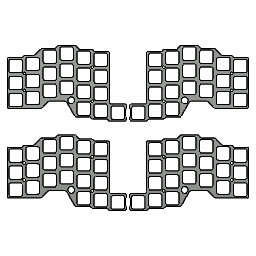
mriya-spacer-fdm-v.1.01 (Autodesk Fusion 360 design; units mm, degrees)
Autodesk Fusion 360 part; units mm, degrees
note: some values were not read from the file. Set by a fixed rule: which sketch regions a step uses.
(part 1 of 2)
sketch "mriya-spacer-fdm" plane through (0, 0, 0) normal (0, 0, 1) x (1, 0, 0)
  arc A0 (-5.2, 2.5932) -> (-4.4, 3.3932) centre (-5.2, 3.3932) ccw construction
  line L0 (-2.1, 1.9932) -> (-2.1, 37.3932) construction
  arc A1 (-3.6, 0.4932) -> (-2.1, 1.9932) centre (-3.6, 1.9932) ccw construction
  line L1 (-36.6, 37.8932) -> (-24.2, 37.8932) construction
  line L2 (-36.6, 23.8932) -> (-24.2, 23.8932) construction
  line L3 (-36.6, 18.8932) -> (-24.2, 18.8932) construction
  line L4 (-36.6, 4.8932) -> (-24.2, 4.8932) construction
  arc A2 (-67.7517, 20.7608) -> (-71.2344, 22.7932) centre (-71.2344, 18.793) ccw construction
  line L5 (-39.0716, 2.7932) -> (-24.0284, 2.7932) construction
  line L6 (-36.6, 42.8932) -> (-24.2, 42.8932) construction
  arc A3 (-56.4, 7.9932) -> (-55.6, 7.1932) centre (-55.6, 7.9932) ccw construction
  arc A4 (-36.6, 18.8932) -> (-37.4, 18.0932) centre (-36.6, 18.0932) ccw construction
  line L7 (-37.4, 18.0932) -> (-37.4, 5.6932) construction
  arc A5 (-40.4858, 3.379) -> (-39.0716, 2.7932) centre (-39.0716, 4.7932) ccw construction
  circle A6 centre (-39.9, 22.5432) radius 1.7
  arc A7 (-20.7, 39.1932) -> (-19.7, 38.1932) centre (-19.7, 39.1932) ccw construction
  line L8 (-3.6, 0.4932) -> (-20.0716, 0.4932) construction
  arc A8 (-17.6, 16.5932) -> (-18.4, 15.7932) centre (-17.6, 15.7932) ccw construction
  line L9 (-17.6, 16.5932) -> (-5.2, 16.5932) construction
  arc A9 (-18.4, 3.3932) -> (-17.6, 2.5932) centre (-17.6, 3.3932) ccw construction
  arc A10 (-2.1, 37.3932) -> (-2.9, 38.1932) centre (-2.9, 37.3932) ccw construction
  arc A11 (-4.4, 15.7932) -> (-5.2, 16.5932) centre (-5.2, 15.7932) ccw construction
  line L10 (-19.7, 38.1932) -> (-2.9, 38.1932) construction
  line L11 (-18.4, 15.7932) -> (-18.4, 3.3932) construction
  line L12 (-17.6, 2.5932) -> (-5.2, 2.5932) construction
  line L13 (-2.8, 14.0932) -> (-2.8, 5.0932)
  line L14 (-4.4, 15.7932) -> (-4.4, 3.3932) construction
  arc A12 (-24.2, 4.8932) -> (-23.4, 5.6932) centre (-24.2, 5.6932) ccw construction
  line L15 (-56.4, 39.3932) -> (-56.4, 26.9932) construction
  line L16 (-42.4, 39.3932) -> (-42.4, 26.9932) construction
  line L17 (-55.6, 40.1932) -> (-43.2, 40.1932) construction
  arc A13 (-36.6, 37.8932) -> (-37.4, 37.0932) centre (-36.6, 37.0932) ccw construction
  arc A14 (-62.2, 30.6932) -> (-61.4, 31.4932) centre (-62.2, 31.4932) ccw construction
  line L18 (-61.4, 43.8932) -> (-61.4, 31.4932) construction
  line L19 (-55.6, 26.1932) -> (-43.2, 26.1932) construction
  line L20 (-55.6, 45.1932) -> (-43.2, 45.1932) construction
  arc A15 (-43.2, 26.1932) -> (-42.4, 26.9932) centre (-43.2, 26.9932) ccw construction
  line L21 (-36.6, 56.8932) -> (-24.2, 56.8932) construction
  arc A16 (-23.4, 56.0932) -> (-24.2, 56.8932) centre (-24.2, 56.0932) ccw construction
  arc A17 (-62.2, 49.6932) -> (-61.4, 50.4932) centre (-62.2, 50.4932) ccw construction
  arc A18 (-36.6, 56.8932) -> (-37.4, 56.0932) centre (-36.6, 56.0932) ccw construction
  arc A19 (-36.6, 75.8932) -> (-37.4, 75.0932) centre (-36.6, 75.0932) ccw construction
  arc A20 (-43.2, 64.1932) -> (-42.4, 64.9932) centre (-43.2, 64.9932) ccw construction
  arc A21 (-42.4, 77.3932) -> (-43.2, 78.1932) centre (-43.2, 77.3932) ccw construction
  line L22 (-42.4, 77.3932) -> (-42.4, 64.9932) construction
  line L23 (-36.6, 75.8932) -> (-24.2, 75.8932) construction
  line L24 (-38.1858, 78.579) -> (-39.3142, 79.7074) construction
  arc A22 (-20.7, 77.1932) -> (-21.5, 77.9932) centre (-21.5, 77.1932) ccw construction
  arc A23 (-38.1858, 78.579) -> (-36.7716, 77.9932) centre (-36.7716, 79.9932) ccw construction
  line L25 (-36.6, 61.8932) -> (-24.2, 61.8932) construction
  arc A24 (-42.4, 58.3932) -> (-43.2, 59.1932) centre (-43.2, 58.3932) ccw construction
  line L26 (-20.7, 39.1932) -> (-20.7, 77.1932) construction
  line L27 (-20.7, 39.1932) -> (-20.7, 76.4932)
  line L28 (-80.4, 59.3932) -> (-80.4, 46.9932) construction
  line L29 (-56.4, 58.3932) -> (-56.4, 45.9932) construction
  line L30 (-37.4, 75.0932) -> (-37.4, 62.6932) construction
  line L31 (-118.4, 49.0932) -> (-118.4, 36.6932) construction
  line L32 (-74.6, 82.6932) -> (-62.2, 82.6932) construction
  circle A25 centre (-39.9, 60.5432) radius 1.7
  arc A26 (-56.4, 64.9932) -> (-55.6, 64.1932) centre (-55.6, 64.9932) ccw construction
  arc A27 (-23.4, 75.0932) -> (-24.2, 75.8932) centre (-24.2, 75.0932) ccw construction
  arc A28 (-37.4, 62.6932) -> (-36.6, 61.8932) centre (-36.6, 62.6932) ccw construction
  line L33 (-99.4, 51.3932) -> (-99.4, 38.9932) construction
  line L34 (-113.4, 51.3932) -> (-113.4, 38.9932) construction
  line L35 (-23.4, 75.0932) -> (-23.4, 62.6932) construction
  arc A29 (-24.2, 61.8932) -> (-23.4, 62.6932) centre (-24.2, 62.6932) ccw construction
  line L36 (-132.4, 49.0932) -> (-132.4, 36.6932) construction
  line L37 (-42.4, 58.3932) -> (-42.4, 45.9932) construction
  line L38 (-23.4, 56.0932) -> (-23.4, 43.6932) construction
  arc A30 (-39.3142, 79.7074) -> (-40.7284, 80.2932) centre (-40.7284, 78.2932) ccw construction
  line L39 (-36.7716, 77.9932) -> (-21.5, 77.9932) construction
  arc A31 (-55.6, 59.1932) -> (-56.4, 58.3932) centre (-55.6, 58.3932) ccw construction
  arc A32 (-54.9858, 80.879) -> (-53.5716, 80.2932) centre (-53.5716, 82.2931) ccw construction
  arc A33 (-55.6, 78.1932) -> (-56.4, 77.3932) centre (-55.6, 77.3932) ccw construction
  line L40 (-56.4, 77.3932) -> (-56.4, 64.9932) construction
  arc A34 (-62.2, 68.6932) -> (-61.4, 69.4932) centre (-62.2, 69.4932) ccw construction
  line L41 (-58.3142, 84.2074) -> (-54.9858, 80.879) construction
  arc A35 (-61.4, 81.8932) -> (-62.2, 82.6932) centre (-62.2, 81.8932) ccw construction
  arc A36 (-58.3142, 84.2074) -> (-59.7284, 84.7932) centre (-59.7284, 82.7932) ccw construction
  line L42 (-74.6, 49.6932) -> (-62.2, 49.6932) construction
  line L43 (-77.0716, 84.7932) -> (-59.7284, 84.7932) construction
  line L44 (-74.6, 68.6932) -> (-62.2, 68.6932) construction
  arc A37 (-61.4, 62.8932) -> (-62.2, 63.6932) centre (-62.2, 62.8932) ccw construction
  line L45 (-74.6, 63.6932) -> (-62.2, 63.6932) construction
  arc A38 (-113.4, 19.9932) -> (-112.6, 19.1932) centre (-112.6, 19.9932) ccw construction
  arc A39 (-119.2, 35.8932) -> (-118.4, 36.6932) centre (-119.2, 36.6932) ccw construction
  arc A40 (-118.4, 30.0932) -> (-119.2, 30.8932) centre (-119.2, 30.0932) ccw construction
  arc A41 (-132.4, 17.6932) -> (-131.6, 16.8932) centre (-131.6, 17.6932) ccw construction
  line L46 (-131.6, 16.8932) -> (-119.2, 16.8932) construction
  arc A42 (-131.6, 30.8932) -> (-132.4, 30.0932) centre (-131.6, 30.0932) ccw construction
  line L47 (-132.4, 30.0932) -> (-132.4, 17.6932) construction
  arc A43 (-119.2, 16.8932) -> (-118.4, 17.6932) centre (-119.2, 17.6932) ccw construction
  arc A44 (-112.6, 33.1932) -> (-113.4, 32.3932) centre (-112.6, 32.3932) ccw construction
  line L48 (-131.6, 30.8932) -> (-119.2, 30.8932) construction
  arc A45 (-134.6, 16.2932) -> (-133.1, 14.7932) centre (-133.1, 16.2932) ccw construction
  line L49 (-131.6, 35.8932) -> (-119.2, 35.8932) construction
  line L50 (-113.4, 32.3932) -> (-113.4, 19.9932) construction
  line L51 (-118.4, 30.0932) -> (-118.4, 17.6932) construction
  line L52 (-112.6, 38.1932) -> (-100.2, 38.1932) construction
  line L53 (-112.6, 33.1932) -> (-100.2, 33.1932) construction
  arc A46 (-132.4, 36.6932) -> (-131.6, 35.8932) centre (-131.6, 36.6932) ccw construction
  arc A47 (-113.4, 38.9932) -> (-112.6, 38.1932) centre (-112.6, 38.9932) ccw construction
  circle A48 centre (-115.9, 34.5432) radius 1.7
  line L54 (-112.6, 19.1932) -> (-100.2, 19.1932) construction
  line L55 (-59.4741, 6.1094) -> (-67.7517, 20.7608) construction
  line L56 (-133.1, 14.7932) -> (-98.1426, 14.7932) construction
  line L57 (-74.6, 44.6932) -> (-62.2, 44.6932) construction
  circle A49 centre (-63.3, 23.4932) radius 3.8
  line L58 (-74.6, 30.6932) -> (-62.2, 30.6932) construction
  circle A50 centre (-5.1, 22.4932) radius 1
  line L59 (-23.4, 18.0932) -> (-23.4, 5.6932) construction
  circle A51 centre (-17.6, 22.4932) radius 1
  arc A52 (-21.4858, 1.079) -> (-20.0716, 0.4932) centre (-20.0716, 2.4932) ccw construction
  arc A53 (-22.6142, 2.2074) -> (-24.0284, 2.7932) centre (-24.0284, 0.7933) ccw construction
  line L60 (-21.4858, 1.079) -> (-22.6142, 2.2074) construction
  arc A54 (-23.4, 18.0932) -> (-24.2, 18.8932) centre (-24.2, 18.0932) ccw construction
  line L61 (-23.4, 37.0932) -> (-23.4, 24.6932) construction
  arc A55 (-1.95, 24.6932) -> (-2.1, 25.1596) centre (-2.75, 24.6932) ccw
  arc A56 (-24.2, 42.8932) -> (-23.4, 43.6932) centre (-24.2, 43.6932) ccw construction
  line L62 (-80.4, 40.3932) -> (-80.4, 27.9932) construction
  arc A57 (-99.4, 32.3932) -> (-100.2, 33.1932) centre (-100.2, 32.3932) ccw construction
  line L63 (-93.6, 27.1932) -> (-81.2, 27.1932) construction
  arc A58 (-94.4, 46.9932) -> (-93.6, 46.1932) centre (-93.6, 46.9932) ccw construction
  arc A59 (-98.1426, 14.7932) -> (-96.0213, 15.6719) centre (-98.1426, 17.7931) ccw construction
  arc A60 (-81.2, 27.1932) -> (-80.4, 27.9932) centre (-81.2, 27.9932) ccw construction
  arc A61 (-93.6, 41.1932) -> (-94.4, 40.3932) centre (-93.6, 40.3932) ccw construction
  arc A62 (-87.6574, 22.7932) -> (-89.7787, 21.9145) centre (-87.6573, 19.7931) ccw construction
  line L64 (-93.6, 41.1932) -> (-81.2, 41.1932) construction
  line L65 (-87.6574, 22.7932) -> (-71.2344, 22.7932) construction
  arc A63 (-37.4, 43.6932) -> (-36.6, 42.8932) centre (-36.6, 43.6932) ccw construction
  arc A64 (-56.4, 26.9932) -> (-55.6, 26.1932) centre (-55.6, 26.9932) ccw construction
  arc A65 (-37.4, 24.6932) -> (-36.6, 23.8932) centre (-36.6, 24.6932) ccw construction
  arc A66 (-42.4, 39.3932) -> (-43.2, 40.1932) centre (-43.2, 39.3932) ccw construction
  arc A67 (-61.4, 43.8932) -> (-62.2, 44.6932) centre (-62.2, 43.8932) ccw construction
  arc A68 (-55.6, 40.1932) -> (-56.4, 39.3932) centre (-55.6, 39.3932) ccw construction
  line L66 (-56.4, 20.3932) -> (-56.4, 7.9932) construction
  line L67 (-55.6, 7.1932) -> (-43.2, 7.1932) construction
  arc A69 (-55.6, 21.1932) -> (-56.4, 20.3932) centre (-55.6, 20.3932) ccw construction
  arc A70 (-43.2, 7.1932) -> (-42.4, 7.9932) centre (-43.2, 7.9932) ccw construction
  arc A71 (-37.4, 5.6932) -> (-36.6, 4.8932) centre (-36.6, 5.6932) ccw construction
  arc A72 (-41.6142, 4.5074) -> (-43.0284, 5.0932) centre (-43.0284, 3.0933) ccw construction
  line L68 (-42.4, 20.3932) -> (-42.4, 7.9932) construction
  line L69 (-43.0284, 5.0932) -> (-57.7328, 5.0932) construction
  line L70 (-40.4858, 3.379) -> (-41.6142, 4.5074) construction
  line L71 (-55.6, 21.1932) -> (-43.2, 21.1932) construction
  arc A73 (-59.4741, 6.1094) -> (-57.7328, 5.0932) centre (-57.7328, 7.0932) ccw construction
  line L72 (-37.4, 37.0932) -> (-37.4, 24.6932) construction
  arc A74 (-56.4, 45.9932) -> (-55.6, 45.1932) centre (-55.6, 45.9932) ccw construction
  arc A75 (-42.4, 20.3932) -> (-43.2, 21.1932) centre (-43.2, 20.3932) ccw construction
  arc A76 (-43.2, 45.1932) -> (-42.4, 45.9932) centre (-43.2, 45.9932) ccw construction
  arc A77 (-81.2, 46.1932) -> (-80.4, 46.9932) centre (-81.2, 46.9932) ccw construction
  line L73 (-99.4, 32.3932) -> (-99.4, 19.9932) construction
  line L74 (-96.0213, 15.6719) -> (-89.7787, 21.9145) construction
  arc A78 (-80.4, 40.3932) -> (-81.2, 41.1932) centre (-81.2, 40.3932) ccw construction
  arc A79 (-100.2, 19.1932) -> (-99.4, 19.9932) centre (-100.2, 19.9932) ccw construction
  line L75 (-93.6, 46.1932) -> (-81.2, 46.1932) construction
  line L76 (-94.4, 40.3932) -> (-94.4, 27.9932) construction
  arc A80 (-100.2, 38.1932) -> (-99.4, 38.9932) centre (-100.2, 38.9932) ccw construction
  arc A81 (-94.4, 27.9932) -> (-93.6, 27.1932) centre (-93.6, 27.9932) ccw construction
  arc A82 (-75.4, 31.4932) -> (-74.6, 30.6932) centre (-74.6, 31.4932) ccw construction
  arc A83 (-74.6, 44.6932) -> (-75.4, 43.8932) centre (-74.6, 43.8932) ccw construction
  line L77 (-75.4, 43.8932) -> (-75.4, 31.4932) construction
  arc A84 (-100.2, 57.1932) -> (-99.4, 57.9932) centre (-100.2, 57.9932) ccw construction
  arc A85 (-75.4, 50.4932) -> (-74.6, 49.6932) centre (-74.6, 50.4932) ccw construction
  arc A86 (-93.6, 60.1932) -> (-94.4, 59.3932) centre (-93.6, 59.3932) ccw construction
  line L78 (-93.6, 65.1932) -> (-81.2, 65.1932) construction
  line L79 (-55.6, 64.1932) -> (-43.2, 64.1932) construction
  circle A87 centre (-115.9, 53.5432) radius 1.7
  line L80 (-106.1426, 73.2932) -> (-115.0716, 73.2932) construction
  line L81 (-61.4, 81.8932) -> (-61.4, 69.4932) construction
  line L82 (-112.6, 52.1932) -> (-100.2, 52.1932) construction
  line L83 (-112.6, 57.1932) -> (-100.2, 57.1932) construction
  line L84 (-112.6, 71.1932) -> (-100.2, 71.1932) construction
  arc A88 (-74.6, 63.6932) -> (-75.4, 62.8932) centre (-74.6, 62.8932) ccw construction
  arc A89 (-94.4, 65.9932) -> (-93.6, 65.1932) centre (-93.6, 65.9932) ccw construction
  arc A90 (-115.0716, 73.2932) -> (-116.4858, 72.7074) centre (-115.0716, 71.2933) ccw construction
  arc A91 (-99.4, 51.3932) -> (-100.2, 52.1932) centre (-100.2, 51.3932) ccw construction
  line L85 (-55.6, 59.1932) -> (-43.2, 59.1932) construction
  arc A92 (-80.4, 59.3932) -> (-81.2, 60.1932) centre (-81.2, 59.3932) ccw construction
  line L86 (-93.6, 60.1932) -> (-81.2, 60.1932) construction
  line L87 (-104.0213, 74.1719) -> (-97.4858, 80.7074) construction
  line L88 (-113.4, 70.3932) -> (-113.4, 57.9932) construction
  arc A93 (-113.4, 57.9932) -> (-112.6, 57.1932) centre (-112.6, 57.9932) ccw construction
  arc A94 (-112.6, 71.1932) -> (-113.4, 70.3932) centre (-112.6, 70.3932) ccw construction
  arc A95 (-81.2, 65.1932) -> (-80.4, 65.9932) centre (-81.2, 65.9932) ccw construction
  line L89 (-53.5716, 80.2932) -> (-40.7284, 80.2932) construction
  line L90 (-55.6, 78.1932) -> (-43.2, 78.1932) construction
  arc A96 (-106.1426, 73.2932) -> (-104.0213, 74.1719) centre (-106.1426, 76.2932) ccw construction
  line L91 (-99.4, 70.3932) -> (-99.4, 57.9932) construction
  arc A97 (-112.6, 52.1932) -> (-113.4, 51.3932) centre (-112.6, 51.3932) ccw construction
  line L92 (-75.4, 62.8932) -> (-75.4, 50.4932) construction
  line L93 (-61.4, 62.8932) -> (-61.4, 50.4932) construction
  line L94 (-78.4858, 84.2074) -> (-80.8142, 81.879) construction
  line L95 (-80.4, 78.3932) -> (-80.4, 65.9932) construction
  arc A98 (-77.0716, 84.7932) -> (-78.4858, 84.2074) centre (-77.0716, 82.7933) ccw construction
  arc A99 (-82.2284, 81.2932) -> (-80.8142, 81.879) centre (-82.2284, 83.2932) ccw construction
  arc A100 (-80.4, 78.3932) -> (-81.2, 79.1932) centre (-81.2, 78.3932) ccw construction
  arc A101 (-74.6, 82.6932) -> (-75.4, 81.8932) centre (-74.6, 81.8932) ccw construction
  line L96 (-132.4, 68.0932) -> (-132.4, 55.6932) construction
  arc A102 (-132.4, 55.6932) -> (-131.6, 54.8932) centre (-131.6, 55.6932) ccw construction
  arc A103 (-131.6, 68.8932) -> (-132.4, 68.0932) centre (-131.6, 68.0932) ccw construction
  arc A104 (-99.4, 70.3932) -> (-100.2, 71.1932) centre (-100.2, 70.3932) ccw construction
  arc A105 (-96.0716, 81.2932) -> (-97.4858, 80.7074) centre (-96.0716, 79.2933) ccw construction
  line L97 (-75.4, 81.8932) -> (-75.4, 69.4932) construction
  arc A106 (-93.6, 79.1932) -> (-94.4, 78.3932) centre (-93.6, 78.3932) ccw construction
  line L98 (-117.6142, 71.579) -> (-116.4858, 72.7074) construction
  line L99 (-131.6, 68.8932) -> (-119.2, 68.8932) construction
  arc A107 (-118.4, 49.0932) -> (-119.2, 49.8932) centre (-119.2, 49.0932) ccw construction
  line L100 (-131.6, 49.8932) -> (-119.2, 49.8932) construction
  arc A108 (-75.4, 69.4932) -> (-74.6, 68.6932) centre (-74.6, 69.4932) ccw construction
  line L101 (-93.6, 79.1932) -> (-81.2, 79.1932) construction
  line L102 (-118.4, 68.0932) -> (-118.4, 55.6932) construction
  line L103 (-96.0716, 81.2932) -> (-82.2284, 81.2932) construction
  line L104 (-131.6, 54.8932) -> (-119.2, 54.8932) construction
  line L105 (-94.4, 78.3932) -> (-94.4, 65.9932) construction
  arc A109 (-118.4, 68.0932) -> (-119.2, 68.8932) centre (-119.2, 68.0932) ccw construction
  arc A110 (-131.6, 49.8932) -> (-132.4, 49.0932) centre (-131.6, 49.0932) ccw construction
  arc A111 (-119.2, 54.8932) -> (-118.4, 55.6932) centre (-119.2, 55.6932) ccw construction
  line L106 (-133.1, 70.9932) -> (-119.0284, 70.9932) construction
  arc A112 (-133.1, 70.9932) -> (-134.6, 69.4932) centre (-133.1, 69.4932) ccw construction
  arc A113 (-119.0284, 70.9932) -> (-117.6142, 71.579) centre (-119.0284, 72.9932) ccw construction
  line L107 (-37.4, 56.0932) -> (-37.4, 43.6932) construction
  line L108 (-134.6, 69.4932) -> (-134.6, 16.2932) construction
  line L109 (-94.4, 59.3932) -> (-94.4, 46.9932) construction
  arc A114 (-23.4, 37.0932) -> (-24.2, 37.8932) centre (-24.2, 37.0932) ccw construction
  arc A115 (-24.2, 23.8932) -> (-23.4, 24.6932) centre (-24.2, 24.6932) ccw construction
  line L110 (-20.7, 21.2432) -> (-20.7, 39.1932)
  line L111 (-130.9, 69.3932) -> (-119.9, 69.3932)
  line L112 (-132.9, 67.3932) -> (-132.9, 56.3932)
  line L113 (-130.9, 54.3932) -> (-119.9, 54.3932)
  line L114 (-117.9, 67.3932) -> (-117.9, 56.3932)
  arc A116 (-59.6047, 6.0356) -> (-57.7328, 4.9432) centre (-57.7328, 7.0932) ccw
  line L115 (-43.0284, 4.9432) -> (-57.7328, 4.9432)
  arc A117 (-41.7203, 4.4013) -> (-43.0284, 4.9432) centre (-43.0284, 3.0933) ccw
  line L116 (-40.5919, 3.2729) -> (-41.7203, 4.4013)
  arc A118 (-40.5919, 3.2729) -> (-39.0716, 2.6432) centre (-39.0716, 4.7932) ccw
  line L117 (-39.0716, 2.6432) -> (-24.0284, 2.6432)
  arc A119 (-22.7203, 2.1013) -> (-24.0284, 2.6432) centre (-24.0284, 0.7933) ccw
  line L118 (-21.5919, 0.9729) -> (-22.7203, 2.1013)
  arc A120 (-21.5919, 0.9729) -> (-20.0716, 0.3432) centre (-20.0716, 2.4932) ccw
  line L119 (-3.6, 0.3432) -> (-20.0716, 0.3432)
  arc A121 (-3.6, 0.3432) -> (-1.95, 1.9932) centre (-3.6, 1.9932) ccw
  line L120 (-36.7716, 78.1432) -> (-22.35, 78.1432)
  arc A122 (-38.0797, 78.6851) -> (-36.7716, 78.1432) centre (-36.7716, 79.9932) ccw
  line L121 (-38.0797, 78.6851) -> (-39.2081, 79.8135)
  arc A123 (-39.2081, 79.8135) -> (-40.7284, 80.4432) centre (-40.7284, 78.2932) ccw
  line L122 (-53.5716, 80.4432) -> (-40.7284, 80.4432)
  arc A124 (-54.8797, 80.9851) -> (-53.5716, 80.4432) centre (-53.5716, 82.2931) ccw
  line L123 (-58.2081, 84.3135) -> (-54.8797, 80.9851)
  arc A125 (-58.2081, 84.3135) -> (-59.7284, 84.9432) centre (-59.7284, 82.7932) ccw
  line L124 (-77.0716, 84.9432) -> (-59.7284, 84.9432)
  arc A126 (-77.0716, 84.9432) -> (-78.5919, 84.3135) centre (-77.0716, 82.7933) ccw
  line L125 (-78.5919, 84.3135) -> (-80.9203, 81.9851)
  arc A127 (-82.2284, 81.4432) -> (-80.9203, 81.9851) centre (-82.2284, 83.2932) ccw
  line L126 (-96.0716, 81.4432) -> (-82.2284, 81.4432)
  arc A128 (-96.0716, 81.4432) -> (-97.5918, 80.8135) centre (-96.0716, 79.2933) ccw
  line L127 (-104.1274, 74.2779) -> (-97.5918, 80.8135)
  arc A129 (-106.1426, 73.4432) -> (-104.1274, 74.2779) centre (-106.1426, 76.2932) ccw
  line L128 (-106.1426, 73.4432) -> (-115.0716, 73.4432)
  arc A130 (-115.0716, 73.4432) -> (-116.5919, 72.8135) centre (-115.0716, 71.2933) ccw
  line L129 (-117.7203, 71.6851) -> (-116.5919, 72.8135)
  arc A131 (-119.0284, 71.1432) -> (-117.7203, 71.6851) centre (-119.0284, 72.9932) ccw
  line L130 (-133.1, 71.1432) -> (-119.0284, 71.1432)
  arc A132 (-133.1, 71.1432) -> (-134.75, 69.4932) centre (-133.1, 69.4932) ccw
  line L131 (-134.75, 69.4932) -> (-134.75, 16.2932)
  arc A133 (-134.75, 16.2932) -> (-133.1, 14.6432) centre (-133.1, 16.2932) ccw
  line L132 (-133.1, 14.6432) -> (-98.1426, 14.6432)
  arc A134 (-98.1426, 14.6432) -> (-95.9152, 15.5658) centre (-98.1426, 17.7931) ccw
  line L133 (-95.9152, 15.5658) -> (-89.6726, 21.8084)
  arc A135 (-87.6574, 22.6432) -> (-89.6726, 21.8084) centre (-87.6573, 19.7931) ccw
  line L134 (-87.6574, 22.6432) -> (-71.2344, 22.6432)
  arc A136 (-67.8823, 20.687) -> (-71.2344, 22.6432) centre (-71.2344, 18.793) ccw
  line L135 (-59.6047, 6.0356) -> (-67.8823, 20.687)
  line L136 (-2.8, 5.0932) -> (-1.95, 5.0932)
  line L137 (-2.8, 14.0932) -> (-1.95, 14.0932)
  line L138 (-1.95, 1.9932) -> (-1.95, 5.0932)
  line L139 (-1.95, 14.0932) -> (-1.95, 17.9432)
  arc A137 (-12.7, 24.1932) -> (-12.7, 20.7932) centre (-12.7, 22.4932) ccw construction
  arc A138 (-10.1, 20.7932) -> (-10.1, 24.1932) centre (-10.1, 22.4932) ccw construction
  line L140 (-12.7, 24.1932) -> (-10.1, 24.1932) construction
  line L141 (-10.1, 20.7932) -> (-12.7, 20.7932) construction
  line L142 (-19.05, 19.5932) -> (-3.6, 19.5932)
  arc A139 (-130.9, 69.3932) -> (-132.9, 67.3932) centre (-130.9, 67.3932) ccw
  arc A140 (-117.9, 67.3932) -> (-119.9, 69.3932) centre (-119.9, 67.3932) ccw
  arc A141 (-132.9, 56.3932) -> (-130.9, 54.3932) centre (-130.9, 56.3932) ccw
  arc A142 (-119.9, 54.3932) -> (-117.9, 56.3932) centre (-119.9, 56.3932) ccw
  arc A143 (-100.9, 56.6932) -> (-98.9, 58.6932) centre (-100.9, 58.6932) ccw
  line L143 (-111.9, 56.6932) -> (-100.9, 56.6932)
  arc A144 (-113.9, 58.6932) -> (-111.9, 56.6932) centre (-111.9, 58.6932) ccw
  line L144 (-113.9, 69.6932) -> (-113.9, 58.6932)
  arc A145 (-111.9, 71.6932) -> (-113.9, 69.6932) centre (-111.9, 69.6932) ccw
  line L145 (-111.9, 71.6932) -> (-100.9, 71.6932)
  arc A146 (-98.9, 69.6932) -> (-100.9, 71.6932) centre (-100.9, 69.6932) ccw
  line L146 (-98.9, 69.6932) -> (-98.9, 58.6932)
  line L147 (-79.9, 77.6932) -> (-79.9, 66.6932)
  arc A147 (-79.9, 77.6932) -> (-81.9, 79.6932) centre (-81.9, 77.6932) ccw
  line L148 (-92.9, 79.6932) -> (-81.9, 79.6932)
  arc A148 (-92.9, 79.6932) -> (-94.9, 77.6932) centre (-92.9, 77.6932) ccw
  line L149 (-94.9, 77.6932) -> (-94.9, 66.6932)
  arc A149 (-94.9, 66.6932) -> (-92.9, 64.6932) centre (-92.9, 66.6932) ccw
  line L150 (-92.9, 64.6932) -> (-81.9, 64.6932)
  arc A150 (-81.9, 64.6932) -> (-79.9, 66.6932) centre (-81.9, 66.6932) ccw
  line L151 (-60.9, 81.1932) -> (-60.9, 70.1932)
  arc A151 (-60.9, 81.1932) -> (-62.9, 83.1932) centre (-62.9, 81.1932) ccw
  line L152 (-73.9, 83.1932) -> (-62.9, 83.1932)
  arc A152 (-73.9, 83.1932) -> (-75.9, 81.1932) centre (-73.9, 81.1932) ccw
  line L153 (-75.9, 81.1932) -> (-75.9, 70.1932)
  arc A153 (-75.9, 70.1932) -> (-73.9, 68.1932) centre (-73.9, 70.1932) ccw
  line L154 (-73.9, 68.1932) -> (-62.9, 68.1932)
  arc A154 (-62.9, 68.1932) -> (-60.9, 70.1932) centre (-62.9, 70.1932) ccw
  line L155 (-41.9, 76.6932) -> (-41.9, 65.6932)
  arc A155 (-41.9, 76.6932) -> (-43.9, 78.6932) centre (-43.9, 76.6932) ccw
  line L156 (-54.9, 78.6932) -> (-43.9, 78.6932)
  arc A156 (-54.9, 78.6932) -> (-56.9, 76.6932) centre (-54.9, 76.6932) ccw
  line L157 (-56.9, 76.6932) -> (-56.9, 65.6932)
  arc A157 (-56.9, 65.6932) -> (-54.9, 63.6932) centre (-54.9, 65.6932) ccw
  line L158 (-54.9, 63.6932) -> (-43.9, 63.6932)
  arc A158 (-43.9, 63.6932) -> (-41.9, 65.6932) centre (-43.9, 65.6932) ccw
  line L159 (-22.9, 74.3932) -> (-22.9, 63.3932)
  arc A159 (-22.9, 74.3932) -> (-24.9, 76.3932) centre (-24.9, 74.3932) ccw
  line L160 (-35.9, 76.3932) -> (-24.9, 76.3932)
  arc A160 (-35.9, 76.3932) -> (-37.9, 74.3932) centre (-35.9, 74.3932) ccw
  line L161 (-37.9, 74.3932) -> (-37.9, 63.3932)
  arc A161 (-37.9, 63.3932) -> (-35.9, 61.3932) centre (-35.9, 63.3932) ccw
  line L162 (-35.9, 61.3932) -> (-24.9, 61.3932)
  arc A162 (-24.9, 61.3932) -> (-22.9, 63.3932) centre (-24.9, 63.3932) ccw
  line L163 (-117.9, 48.3932) -> (-117.9, 37.3932)
  arc A163 (-117.9, 48.3932) -> (-119.9, 50.3932) centre (-119.9, 48.3932) ccw
  line L164 (-130.9, 50.3932) -> (-119.9, 50.3932)
  arc A164 (-130.9, 50.3932) -> (-132.9, 48.3932) centre (-130.9, 48.3932) ccw
  line L165 (-132.9, 48.3932) -> (-132.9, 37.3932)
  arc A165 (-132.9, 37.3932) -> (-130.9, 35.3932) centre (-130.9, 37.3932) ccw
  line L166 (-130.9, 35.3932) -> (-119.9, 35.3932)
  arc A166 (-119.9, 35.3932) -> (-117.9, 37.3932) centre (-119.9, 37.3932) ccw
  line L167 (-98.9, 50.6932) -> (-98.9, 39.6932)
  arc A167 (-98.9, 50.6932) -> (-100.9, 52.6932) centre (-100.9, 50.6932) ccw
  line L168 (-111.9, 52.6932) -> (-100.9, 52.6932)
  arc A168 (-111.9, 52.6932) -> (-113.9, 50.6932) centre (-111.9, 50.6932) ccw
  line L169 (-113.9, 50.6932) -> (-113.9, 39.6932)
  arc A169 (-113.9, 39.6932) -> (-111.9, 37.6932) centre (-111.9, 39.6932) ccw
  arc A170 (-100.9, 37.6932) -> (-98.9, 39.6932) centre (-100.9, 39.6932) ccw
  line L170 (-111.9, 37.6932) -> (-100.9, 37.6932)
  line L171 (-79.9, 58.6932) -> (-79.9, 47.6932)
  arc A171 (-79.9, 58.6932) -> (-81.9, 60.6932) centre (-81.9, 58.6932) ccw
  line L172 (-92.9, 60.6932) -> (-81.9, 60.6932)
  arc A172 (-92.9, 60.6932) -> (-94.9, 58.6932) centre (-92.9, 58.6932) ccw
  line L173 (-94.9, 58.6932) -> (-94.9, 47.6932)
  arc A173 (-94.9, 47.6932) -> (-92.9, 45.6932) centre (-92.9, 47.6932) ccw
  arc A174 (-81.9, 45.6932) -> (-79.9, 47.6932) centre (-81.9, 47.6932) ccw
  line L174 (-92.9, 45.6932) -> (-81.9, 45.6932)
  line L175 (-60.9, 62.1932) -> (-60.9, 51.1932)
  arc A175 (-60.9, 62.1932) -> (-62.9, 64.1932) centre (-62.9, 62.1932) ccw
  line L176 (-73.9, 64.1932) -> (-62.9, 64.1932)
  arc A176 (-73.9, 64.1932) -> (-75.9, 62.1932) centre (-73.9, 62.1932) ccw
  line L177 (-75.9, 62.1932) -> (-75.9, 51.1932)
  arc A177 (-75.9, 51.1932) -> (-73.9, 49.1932) centre (-73.9, 51.1932) ccw
  arc A178 (-62.9, 49.1932) -> (-60.9, 51.1932) centre (-62.9, 51.1932) ccw
  line L178 (-73.9, 49.1932) -> (-62.9, 49.1932)
  line L179 (-41.9, 57.6932) -> (-41.9, 46.6932)
  arc A179 (-41.9, 57.6932) -> (-43.9, 59.6932) centre (-43.9, 57.6932) ccw
  line L180 (-54.9, 59.6932) -> (-43.9, 59.6932)
  arc A180 (-54.9, 59.6932) -> (-56.9, 57.6932) centre (-54.9, 57.6932) ccw
  line L181 (-56.9, 57.6932) -> (-56.9, 46.6932)
  arc A181 (-56.9, 46.6932) -> (-54.9, 44.6932) centre (-54.9, 46.6932) ccw
  arc A182 (-43.9, 44.6932) -> (-41.9, 46.6932) centre (-43.9, 46.6932) ccw
  line L182 (-54.9, 44.6932) -> (-43.9, 44.6932)
  line L183 (-22.9, 55.3932) -> (-22.9, 44.3932)
  arc A183 (-22.9, 55.3932) -> (-24.9, 57.3932) centre (-24.9, 55.3932) ccw
  line L184 (-35.9, 57.3932) -> (-24.9, 57.3932)
  arc A184 (-35.9, 57.3932) -> (-37.9, 55.3932) centre (-35.9, 55.3932) ccw
  line L185 (-37.9, 55.3932) -> (-37.9, 44.3932)
  arc A185 (-37.9, 44.3932) -> (-35.9, 42.3932) centre (-35.9, 44.3932) ccw
  arc A186 (-24.9, 42.3932) -> (-22.9, 44.3932) centre (-24.9, 44.3932) ccw
  line L186 (-35.9, 42.3932) -> (-24.9, 42.3932)
  line L187 (-98.9, 31.6932) -> (-98.9, 20.6932)
  arc A187 (-98.9, 31.6932) -> (-100.9, 33.6932) centre (-100.9, 31.6932) ccw
  line L188 (-111.9, 33.6932) -> (-100.9, 33.6932)
  arc A188 (-111.9, 33.6932) -> (-113.9, 31.6932) centre (-111.9, 31.6932) ccw
  line L189 (-113.9, 31.6932) -> (-113.9, 20.6932)
  arc A189 (-113.9, 20.6932) -> (-111.9, 18.6932) centre (-111.9, 20.6932) ccw
  line L190 (-111.9, 18.6932) -> (-100.9, 18.6932)
  arc A190 (-100.9, 18.6932) -> (-98.9, 20.6932) centre (-100.9, 20.6932) ccw
  line L191 (-117.9, 29.3932) -> (-117.9, 18.3932)
  arc A191 (-117.9, 29.3932) -> (-119.9, 31.3932) centre (-119.9, 29.3932) ccw
  line L192 (-130.9, 31.3932) -> (-119.9, 31.3932)
  arc A192 (-130.9, 31.3932) -> (-132.9, 29.3932) centre (-130.9, 29.3932) ccw
  line L193 (-132.9, 29.3932) -> (-132.9, 18.3932)
  arc A193 (-132.9, 18.3932) -> (-130.9, 16.3932) centre (-130.9, 18.3932) ccw
  arc A194 (-119.9, 16.3932) -> (-117.9, 18.3932) centre (-119.9, 18.3932) ccw
  line L194 (-130.9, 16.3932) -> (-119.9, 16.3932)
  line L195 (-79.9, 39.6932) -> (-79.9, 28.6932)
  arc A195 (-79.9, 39.6932) -> (-81.9, 41.6932) centre (-81.9, 39.6932) ccw
  line L196 (-92.9, 41.6932) -> (-81.9, 41.6932)
  arc A196 (-92.9, 41.6932) -> (-94.9, 39.6932) centre (-92.9, 39.6932) ccw
  line L197 (-94.9, 39.6932) -> (-94.9, 28.6932)
  arc A197 (-94.9, 28.6932) -> (-92.9, 26.6932) centre (-92.9, 28.6932) ccw
  arc A198 (-81.9, 26.6932) -> (-79.9, 28.6932) centre (-81.9, 28.6932) ccw
  line L198 (-92.9, 26.6932) -> (-81.9, 26.6932)
  line L199 (-60.9, 43.1932) -> (-60.9, 32.1932)
  arc A199 (-60.9, 43.1932) -> (-62.9, 45.1932) centre (-62.9, 43.1932) ccw
  line L200 (-73.9, 45.1932) -> (-62.9, 45.1932)
  arc A200 (-73.9, 45.1932) -> (-75.9, 43.1932) centre (-73.9, 43.1932) ccw
  line L201 (-75.9, 43.1932) -> (-75.9, 32.1932)
  arc A201 (-75.9, 32.1932) -> (-73.9, 30.1932) centre (-73.9, 32.1932) ccw
  arc A202 (-62.9, 30.1932) -> (-60.9, 32.1932) centre (-62.9, 32.1932) ccw
  line L202 (-73.9, 30.1932) -> (-62.9, 30.1932)
  line L203 (-41.9, 38.6932) -> (-41.9, 27.6932)
  arc A203 (-41.9, 38.6932) -> (-43.9, 40.6932) centre (-43.9, 38.6932) ccw
  line L204 (-54.9, 40.6932) -> (-43.9, 40.6932)
  arc A204 (-54.9, 40.6932) -> (-56.9, 38.6932) centre (-54.9, 38.6932) ccw
  line L205 (-56.9, 38.6932) -> (-56.9, 27.6932)
  arc A205 (-56.9, 27.6932) -> (-54.9, 25.6932) centre (-54.9, 27.6932) ccw
  arc A206 (-43.9, 25.6932) -> (-41.9, 27.6932) centre (-43.9, 27.6932) ccw
  line L206 (-54.9, 25.6932) -> (-43.9, 25.6932)
  line L207 (-22.9, 36.3932) -> (-22.9, 25.3932)
  arc A207 (-22.9, 36.3932) -> (-24.9, 38.3932) centre (-24.9, 36.3932) ccw
  line L208 (-35.9, 38.3932) -> (-24.9, 38.3932)
  arc A208 (-35.9, 38.3932) -> (-37.9, 36.3932) centre (-35.9, 36.3932) ccw
  line L209 (-37.9, 36.3932) -> (-37.9, 25.3932)
  arc A209 (-37.9, 25.3932) -> (-35.9, 23.3932) centre (-35.9, 25.3932) ccw
  arc A210 (-24.9, 23.3932) -> (-22.9, 25.3932) centre (-24.9, 25.3932) ccw
  line L210 (-35.9, 23.3932) -> (-24.9, 23.3932)
  line L211 (-41.9, 19.6932) -> (-41.9, 8.6932)
  arc A211 (-41.9, 19.6932) -> (-43.9, 21.6932) centre (-43.9, 19.6932) ccw
  line L212 (-54.9, 21.6932) -> (-43.9, 21.6932)
  arc A212 (-54.9, 21.6932) -> (-56.9, 19.6932) centre (-54.9, 19.6932) ccw
  line L213 (-56.9, 19.6932) -> (-56.9, 8.6932)
  arc A213 (-56.9, 8.6932) -> (-54.9, 6.6932) centre (-54.9, 8.6932) ccw
  line L214 (-54.9, 6.6932) -> (-43.9, 6.6932)
  arc A214 (-43.9, 6.6932) -> (-41.9, 8.6932) centre (-43.9, 8.6932) ccw
  line L215 (-22.9, 17.3932) -> (-22.9, 6.3932)
  arc A215 (-22.9, 17.3932) -> (-24.9, 19.3932) centre (-24.9, 17.3932) ccw
  line L216 (-35.9, 19.3932) -> (-24.9, 19.3932)
  arc A216 (-35.9, 19.3932) -> (-37.9, 17.3932) centre (-35.9, 17.3932) ccw
  line L217 (-37.9, 17.3932) -> (-37.9, 6.3932)
  arc A217 (-37.9, 6.3932) -> (-35.9, 4.3932) centre (-35.9, 6.3932) ccw
  arc A218 (-24.9, 4.3932) -> (-22.9, 6.3932) centre (-24.9, 6.3932) ccw
  line L218 (-35.9, 4.3932) -> (-24.9, 4.3932)
  line L219 (-4, 15.2932) -> (-4, 3.8932)
  line L220 (-16.9, 17.0932) -> (-5.8, 17.0932)
  arc A219 (-16.9, 17.0932) -> (-18.9, 15.0932) centre (-16.9, 15.0932) ccw
  line L221 (-18.9, 15.0932) -> (-18.9, 4.0932)
  arc A220 (-18.9, 4.0932) -> (-16.9, 2.0932) centre (-16.9, 4.0932) ccw
  line L222 (-16.9, 2.0932) -> (-5.8, 2.0932)
  arc A221 (-4, 15.2932) -> (-5.8, 17.0932) centre (-5.8, 15.2932) ccw
  arc A222 (-5.8, 2.0932) -> (-4, 3.8932) centre (-5.8, 3.8932) ccw
  circle A223 centre (-11.4, 22.4932) radius 1.15 construction
  circle A224 centre (-63.3, 23.4932) radius 1.5 construction
  circle A225 centre (-5.1, 35.1932) radius 1.15 construction
  circle A226 centre (-5.1, 35.1932) radius 2.1 construction
  arc A227 (-20.7, 76.4932) -> (-22.35, 78.1432) centre (-22.35, 76.4932) ccw
  arc A228 (-1.95, 17.9432) -> (-3.6, 19.5932) centre (-3.6, 17.9432) ccw
  arc A229 (-20.7, 21.2432) -> (-19.05, 19.5932) centre (-19.05, 21.2432) ccw
  line L223 (-43.0284, 104.9432) -> (-57.7328, 104.9432)
  line L224 (-41.9, 119.6932) -> (-41.9, 108.6932)
  arc A230 (-36.6, 118.8932) -> (-37.4, 118.0932) centre (-36.6, 118.0932) ccw construction
  arc A231 (-43.2, 107.1932) -> (-42.4, 107.9932) centre (-43.2, 107.9932) ccw construction
  arc A232 (-42.4, 120.3932) -> (-43.2, 121.1932) centre (-43.2, 120.3932) ccw construction
  arc A233 (-56.9, 108.6932) -> (-54.9, 106.6932) centre (-54.9, 108.6932) ccw
  arc A234 (-37.9, 106.3932) -> (-35.9, 104.3932) centre (-35.9, 106.3932) ccw
  arc A235 (-43.9, 125.6932) -> (-41.9, 127.6932) centre (-43.9, 127.6932) ccw
  arc A236 (-55.6, 140.1932) -> (-56.4, 139.3932) centre (-55.6, 139.3932) ccw construction
  arc A237 (-56.9, 127.6932) -> (-54.9, 125.6932) centre (-54.9, 127.6932) ccw
  line L225 (-56.9, 138.6932) -> (-56.9, 127.6932)
  arc A238 (-37.4, 124.6932) -> (-36.6, 123.8932) centre (-36.6, 124.6932) ccw construction
  line L226 (-56.4, 139.3932) -> (-56.4, 126.9932) construction
  arc A239 (-56.4, 126.9932) -> (-55.6, 126.1932) centre (-55.6, 126.9932) ccw construction
  line L227 (-54.9, 125.6932) -> (-43.9, 125.6932)
  line L228 (-55.6, 126.1932) -> (-43.2, 126.1932) construction
  arc A240 (-35.9, 138.3932) -> (-37.9, 136.3932) centre (-35.9, 136.3932) ccw
  arc A241 (-43.2, 126.1932) -> (-42.4, 126.9932) centre (-43.2, 126.9932) ccw construction
  arc A242 (-54.9, 140.6932) -> (-56.9, 138.6932) centre (-54.9, 138.6932) ccw
  line L229 (-37.9, 136.3932) -> (-37.9, 125.3932)
  line L230 (-55.6, 140.1932) -> (-43.2, 140.1932) construction
  line L231 (-54.9, 140.6932) -> (-43.9, 140.6932)
  arc A243 (-43.9, 106.6932) -> (-41.9, 108.6932) centre (-43.9, 108.6932) ccw
  line L232 (-37.4, 118.0932) -> (-37.4, 105.6932) construction
  line L233 (-42.4, 120.3932) -> (-42.4, 107.9932) construction
  line L234 (-37.9, 117.3932) -> (-37.9, 106.3932)
  line L235 (-54.9, 106.6932) -> (-43.9, 106.6932)
  arc A244 (-40.4858, 103.379) -> (-39.0716, 102.7932) centre (-39.0716, 104.7932) ccw construction
  arc A245 (-55.6, 121.1932) -> (-56.4, 120.3932) centre (-55.6, 120.3932) ccw construction
  line L236 (-40.5919, 103.2729) -> (-41.7203, 104.4013)
  arc A246 (-59.4741, 106.1094) -> (-57.7328, 105.0932) centre (-57.7328, 107.0932) ccw construction
  arc A247 (-40.5919, 103.2729) -> (-39.0716, 102.6432) centre (-39.0716, 104.7932) ccw
  arc A248 (-24.2, 123.8932) -> (-23.4, 124.6932) centre (-24.2, 124.6932) ccw construction
  circle A249 centre (-5.1, 135.1932) radius 1.15 construction
  circle A250 centre (-11.4, 122.4932) radius 1.15 construction
  line L237 (-19.7, 138.1932) -> (-2.9, 138.1932) construction
  arc A251 (-1.95, 124.6932) -> (-2.1, 125.1596) centre (-2.75, 124.6932) ccw
  line L238 (-23.4, 137.0932) -> (-23.4, 124.6932) construction
  line L239 (-12.7, 124.1932) -> (-10.1, 124.1932) construction
  arc A252 (-23.4, 137.0932) -> (-24.2, 137.8932) centre (-24.2, 137.0932) ccw construction
  circle A253 centre (-5.1, 135.1932) radius 2.1 construction
  arc A254 (-24.9, 123.3932) -> (-22.9, 125.3932) centre (-24.9, 125.3932) ccw
  circle A255 centre (-5.1, 122.4932) radius 1 construction
  arc A256 (-2.1, 137.3932) -> (-2.9, 138.1932) centre (-2.9, 137.3932) ccw construction
  circle A257 centre (-17.6, 122.4932) radius 1 construction
  line L240 (-22.9, 136.3932) -> (-22.9, 125.3932)
  line L241 (-20.7, 121.2432) -> (-20.7, 139.1932)
  arc A258 (-22.9, 136.3932) -> (-24.9, 138.3932) centre (-24.9, 136.3932) ccw
  arc A259 (-20.7, 139.1932) -> (-19.7, 138.1932) centre (-19.7, 139.1932) ccw construction
  line L242 (-18.9, 115.0932) -> (-18.9, 104.0932)
  arc A260 (-20.7, 121.2432) -> (-19.05, 119.5932) centre (-19.05, 121.2432) ccw
  line L243 (-22.9, 117.3932) -> (-22.9, 106.3932)
  line L244 (-21.5919, 100.9729) -> (-22.7203, 102.1013)
  arc A261 (-18.9, 104.0932) -> (-16.9, 102.0932) centre (-16.9, 104.0932) ccw
  line L245 (-19.05, 119.5932) -> (-3.6, 119.5932)
  arc A262 (-24.2, 104.8932) -> (-23.4, 105.6932) centre (-24.2, 105.6932) ccw construction
  line L246 (-16.9, 102.0932) -> (-5.8, 102.0932)
  arc A263 (-12.7, 124.1932) -> (-12.7, 120.7932) centre (-12.7, 122.4932) ccw construction
  line L247 (-17.6, 116.5932) -> (-5.2, 116.5932) construction
  line L248 (-3.6, 100.4932) -> (-20.0716, 100.4932) construction
  arc A264 (-22.9, 117.3932) -> (-24.9, 119.3932) centre (-24.9, 117.3932) ccw
  line L249 (-21.4858, 101.079) -> (-22.6142, 102.2074) construction
  line L250 (-16.9, 117.0932) -> (-5.8, 117.0932)
  line L251 (-3.6, 100.3432) -> (-20.0716, 100.3432)
  line L252 (-17.6, 102.5932) -> (-5.2, 102.5932) construction
  arc A265 (-21.4858, 101.079) -> (-20.0716, 100.4932) centre (-20.0716, 102.4932) ccw construction
  line L253 (-2.1, 101.9932) -> (-2.1, 137.3932) construction
  arc A266 (-10.1, 120.7932) -> (-10.1, 124.1932) centre (-10.1, 122.4932) ccw construction
  arc A267 (-16.9, 117.0932) -> (-18.9, 115.0932) centre (-16.9, 115.0932) ccw
  arc A268 (-17.6, 116.5932) -> (-18.4, 115.7932) centre (-17.6, 115.7932) ccw construction
  line L254 (-23.4, 118.0932) -> (-23.4, 105.6932) construction
  arc A269 (-23.4, 118.0932) -> (-24.2, 118.8932) centre (-24.2, 118.0932) ccw construction
  arc A270 (-21.5919, 100.9729) -> (-20.0716, 100.3432) centre (-20.0716, 102.4932) ccw
  line L255 (-4, 115.2932) -> (-4, 103.8932)
  line L256 (-1.95, 101.9932) -> (-1.95, 105.0932)
  arc A271 (-18.4, 103.3932) -> (-17.6, 102.5932) centre (-17.6, 103.3932) ccw construction
  arc A272 (-22.6142, 102.2074) -> (-24.0284, 102.7932) centre (-24.0284, 100.7933) ccw construction
  line L257 (-18.4, 115.7932) -> (-18.4, 103.3932) construction
  line L258 (-2.8, 114.0932) -> (-2.8, 105.0932)
  arc A273 (-22.7203, 102.1013) -> (-24.0284, 102.6432) centre (-24.0284, 100.7933) ccw
  arc A274 (-24.9, 104.3932) -> (-22.9, 106.3932) centre (-24.9, 106.3932) ccw
  line L259 (-1.95, 114.0932) -> (-1.95, 117.9432)
  line L260 (-2.8, 114.0932) -> (-1.95, 114.0932)
  line L261 (-2.8, 105.0932) -> (-1.95, 105.0932)
  line L262 (-10.1, 120.7932) -> (-12.7, 120.7932) construction
  line L263 (-4.4, 115.7932) -> (-4.4, 103.3932) construction
  arc A275 (-4.4, 115.7932) -> (-5.2, 116.5932) centre (-5.2, 115.7932) ccw construction
  arc A276 (-5.2, 102.5932) -> (-4.4, 103.3932) centre (-5.2, 103.3932) ccw construction
  arc A277 (-3.6, 100.3432) -> (-1.95, 101.9932) centre (-3.6, 101.9932) ccw
  arc A278 (-4, 115.2932) -> (-5.8, 117.0932) centre (-5.8, 115.2932) ccw
  arc A279 (-1.95, 117.9432) -> (-3.6, 119.5932) centre (-3.6, 117.9432) ccw
  arc A280 (-5.8, 102.0932) -> (-4, 103.8932) centre (-5.8, 103.8932) ccw
  arc A281 (-3.6, 100.4932) -> (-2.1, 101.9932) centre (-3.6, 101.9932) ccw construction
  arc A282 (-42.4, 139.3932) -> (-43.2, 140.1932) centre (-43.2, 139.3932) ccw construction
  arc A283 (-62.2, 130.6932) -> (-61.4, 131.4932) centre (-62.2, 131.4932) ccw construction
  arc A284 (-41.9, 138.6932) -> (-43.9, 140.6932) centre (-43.9, 138.6932) ccw
  line L264 (-37.4, 137.0932) -> (-37.4, 124.6932) construction
  line L265 (-42.4, 139.3932) -> (-42.4, 126.9932) construction
  arc A285 (-36.6, 137.8932) -> (-37.4, 137.0932) centre (-36.6, 137.0932) ccw construction
  arc A286 (-62.9, 130.1932) -> (-60.9, 132.1932) centre (-62.9, 132.1932) ccw
  line L266 (-41.9, 138.6932) -> (-41.9, 127.6932)
  line L267 (-61.4, 162.8932) -> (-61.4, 150.4932) construction
  arc A287 (-41.9, 157.6932) -> (-43.9, 159.6932) centre (-43.9, 157.6932) ccw
  line L268 (-56.9, 157.6932) -> (-56.9, 146.6932)
  line L269 (-55.6, 159.1932) -> (-43.2, 159.1932) construction
  arc A288 (-43.2, 164.1932) -> (-42.4, 164.9932) centre (-43.2, 164.9932) ccw construction
  arc A289 (-43.9, 144.6932) -> (-41.9, 146.6932) centre (-43.9, 146.6932) ccw
  arc A290 (-62.2, 149.6932) -> (-61.4, 150.4932) centre (-62.2, 150.4932) ccw construction
  line L270 (-55.6, 145.1932) -> (-43.2, 145.1932) construction
  arc A291 (-60.9, 162.1932) -> (-62.9, 164.1932) centre (-62.9, 162.1932) ccw
  arc A292 (-61.4, 162.8932) -> (-62.2, 163.6932) centre (-62.2, 162.8932) ccw construction
  arc A293 (-61.4, 143.8932) -> (-62.2, 144.6932) centre (-62.2, 143.8932) ccw construction
  arc A294 (-56.9, 165.6932) -> (-54.9, 163.6932) centre (-54.9, 165.6932) ccw
  arc A295 (-56.4, 164.9932) -> (-55.6, 164.1932) centre (-55.6, 164.9932) ccw construction
  line L271 (-56.4, 158.3932) -> (-56.4, 145.9932) construction
  line L272 (-55.6, 164.1932) -> (-43.2, 164.1932) construction
  line L273 (-54.9, 144.6932) -> (-43.9, 144.6932)
  arc A296 (-62.9, 149.1932) -> (-60.9, 151.1932) centre (-62.9, 151.1932) ccw
  arc A297 (-55.6, 159.1932) -> (-56.4, 158.3932) centre (-55.6, 158.3932) ccw construction
  arc A298 (-54.9858, 180.879) -> (-53.5716, 180.2932) centre (-53.5716, 182.2931) ccw construction
  arc A299 (-56.4, 145.9932) -> (-55.6, 145.1932) centre (-55.6, 145.9932) ccw construction
  arc A300 (-56.9, 146.6932) -> (-54.9, 144.6932) centre (-54.9, 146.6932) ccw
  arc A301 (-58.3142, 184.2074) -> (-59.7284, 184.7932) centre (-59.7284, 182.7932) ccw construction
  arc A302 (-54.8797, 180.9851) -> (-53.5716, 180.4432) centre (-53.5716, 182.2931) ccw
  arc A303 (-42.4, 158.3932) -> (-43.2, 159.1932) centre (-43.2, 158.3932) ccw construction
  line L274 (-41.9, 157.6932) -> (-41.9, 146.6932)
  line L275 (-37.9, 155.3932) -> (-37.9, 144.3932)
  line L276 (-36.6, 156.8932) -> (-24.2, 156.8932) construction
  line L277 (-35.9, 142.3932) -> (-24.9, 142.3932)
  arc A304 (-24.9, 161.3932) -> (-22.9, 163.3932) centre (-24.9, 163.3932) ccw
  line L278 (-23.4, 156.0932) -> (-23.4, 143.6932) construction
  arc A305 (-35.9, 157.3932) -> (-37.9, 155.3932) centre (-35.9, 155.3932) ccw
  arc A306 (-37.9, 144.3932) -> (-35.9, 142.3932) centre (-35.9, 144.3932) ccw
  line L279 (-35.9, 157.3932) -> (-24.9, 157.3932)
  arc A307 (-24.2, 161.8932) -> (-23.4, 162.6932) centre (-24.2, 162.6932) ccw construction
  arc A308 (-24.2, 142.8932) -> (-23.4, 143.6932) centre (-24.2, 143.6932) ccw construction
  circle A309 centre (-39.9, 160.5432) radius 1.5
  line L280 (-36.6, 161.8932) -> (-24.2, 161.8932) construction
  arc A310 (-37.4, 143.6932) -> (-36.6, 142.8932) centre (-36.6, 143.6932) ccw construction
  arc A311 (-37.9, 163.3932) -> (-35.9, 161.3932) centre (-35.9, 163.3932) ccw
  arc A312 (-23.4, 156.0932) -> (-24.2, 156.8932) centre (-24.2, 156.0932) ccw construction
  arc A313 (-22.9, 155.3932) -> (-24.9, 157.3932) centre (-24.9, 155.3932) ccw
  line L281 (-36.6, 142.8932) -> (-24.2, 142.8932) construction
  line L282 (-35.9, 161.3932) -> (-24.9, 161.3932)
  line L283 (-37.4, 156.0932) -> (-37.4, 143.6932) construction
  arc A314 (-60.9, 143.1932) -> (-62.9, 145.1932) centre (-62.9, 143.1932) ccw
  line L284 (-60.9, 162.1932) -> (-60.9, 151.1932)
  line L285 (-42.4, 158.3932) -> (-42.4, 145.9932) construction
  arc A315 (-54.9, 159.6932) -> (-56.9, 157.6932) centre (-54.9, 157.6932) ccw
  arc A316 (-43.9, 163.6932) -> (-41.9, 165.6932) centre (-43.9, 165.6932) ccw
  line L286 (-22.9, 155.3932) -> (-22.9, 144.3932)
  arc A317 (-43.2, 145.1932) -> (-42.4, 145.9932) centre (-43.2, 145.9932) ccw construction
  arc A318 (-37.4, 162.6932) -> (-36.6, 161.8932) centre (-36.6, 162.6932) ccw construction
  arc A319 (-36.6, 156.8932) -> (-37.4, 156.0932) centre (-36.6, 156.0932) ccw construction
  arc A320 (-24.9, 142.3932) -> (-22.9, 144.3932) centre (-24.9, 144.3932) ccw
  line L287 (-54.9, 163.6932) -> (-43.9, 163.6932)
  line L288 (-54.9, 159.6932) -> (-43.9, 159.6932)
  arc A321 (-106.1426, 173.2932) -> (-104.0213, 174.1719) centre (-106.1426, 176.2932) ccw construction
  line L289 (-130.9, 169.3932) -> (-119.9, 169.3932)
  line L290 (-133.1, 171.1432) -> (-119.0284, 171.1432)
  line L291 (-130.9, 150.3932) -> (-119.9, 150.3932)
  arc A322 (-133.1, 171.1432) -> (-134.75, 169.4932) centre (-133.1, 169.4932) ccw
  line L292 (-131.6, 154.8932) -> (-119.2, 154.8932) construction
  arc A323 (-130.9, 150.3932) -> (-132.9, 148.3932) centre (-130.9, 148.3932) ccw
  line L293 (-132.9, 167.3932) -> (-132.9, 156.3932)
  arc A324 (-130.9, 169.3932) -> (-132.9, 167.3932) centre (-130.9, 167.3932) ccw
  line L294 (-106.1426, 173.2932) -> (-115.0716, 173.2932) construction
  arc A325 (-113.4, 157.9932) -> (-112.6, 157.1932) centre (-112.6, 157.9932) ccw construction
  line L295 (-131.6, 168.8932) -> (-119.2, 168.8932) construction
  arc A326 (-112.6, 152.1932) -> (-113.4, 151.3932) centre (-112.6, 151.3932) ccw construction
  arc A327 (-133.1, 170.9932) -> (-134.6, 169.4932) centre (-133.1, 169.4932) ccw construction
  line L296 (-131.6, 149.8932) -> (-119.2, 149.8932) construction
  line L297 (-132.4, 168.0932) -> (-132.4, 155.6932) construction
  arc A328 (-131.6, 168.8932) -> (-132.4, 168.0932) centre (-131.6, 168.0932) ccw construction
  line L298 (-113.4, 132.3932) -> (-113.4, 119.9932) construction
  line L299 (-130.9, 131.3932) -> (-119.9, 131.3932)
  arc A329 (-113.9, 139.6932) -> (-111.9, 137.6932) centre (-111.9, 139.6932) ccw
  line L300 (-111.9, 133.6932) -> (-100.9, 133.6932)
  arc A330 (-132.9, 118.3932) -> (-130.9, 116.3932) centre (-130.9, 118.3932) ccw
  line L301 (-133.1, 114.7932) -> (-98.1426, 114.7932) construction
  arc A331 (-132.4, 117.6932) -> (-131.6, 116.8932) centre (-131.6, 117.6932) ccw construction
  line L302 (-112.6, 171.1932) -> (-100.2, 171.1932) construction
  line L303 (-111.9, 171.6932) -> (-100.9, 171.6932)
  line L304 (-130.9, 135.3932) -> (-119.9, 135.3932)
  line L305 (-112.6, 133.1932) -> (-100.2, 133.1932) construction
  line L306 (-131.6, 130.8932) -> (-119.2, 130.8932) construction
  arc A332 (-134.6, 116.2932) -> (-133.1, 114.7932) centre (-133.1, 116.2932) ccw construction
  line L307 (-74.6, 168.6932) -> (-62.2, 168.6932) construction
  line L308 (-112.6, 138.1932) -> (-100.2, 138.1932) construction
  arc A333 (-119.9, 116.3932) -> (-117.9, 118.3932) centre (-119.9, 118.3932) ccw
  line L309 (-117.9, 129.3932) -> (-117.9, 118.3932)
  line L310 (-112.6, 119.1932) -> (-100.2, 119.1932) construction
  line L311 (-112.6, 152.1932) -> (-100.2, 152.1932) construction
  line L312 (-104.0213, 174.1719) -> (-97.4858, 180.7074) construction
  line L313 (-111.9, 137.6932) -> (-100.9, 137.6932)
  arc A334 (-132.9, 137.3932) -> (-130.9, 135.3932) centre (-130.9, 137.3932) ccw
  line L314 (-112.6, 157.1932) -> (-100.2, 157.1932) construction
  line L315 (-104.1274, 174.2779) -> (-97.5918, 180.8135)
  line L316 (-111.9, 118.6932) -> (-100.9, 118.6932)
  arc A335 (-118.4, 130.0932) -> (-119.2, 130.8932) centre (-119.2, 130.0932) ccw construction
  line L317 (-111.9, 152.6932) -> (-100.9, 152.6932)
  arc A336 (-112.6, 133.1932) -> (-113.4, 132.3932) centre (-112.6, 132.3932) ccw construction
  line L318 (-73.9, 145.1932) -> (-62.9, 145.1932)
  arc A337 (-117.9, 129.3932) -> (-119.9, 131.3932) centre (-119.9, 129.3932) ccw
  line L319 (-133.1, 114.6432) -> (-98.1426, 114.6432)
  line L320 (-111.9, 156.6932) -> (-100.9, 156.6932)
  line L321 (-131.6, 135.8932) -> (-119.2, 135.8932) construction
  line L322 (-132.9, 148.3932) -> (-132.9, 137.3932)
  arc A338 (-119.9, 154.3932) -> (-117.9, 156.3932) centre (-119.9, 156.3932) ccw
  arc A339 (-113.9, 158.6932) -> (-111.9, 156.6932) centre (-111.9, 158.6932) ccw
  arc A340 (-119.9, 135.3932) -> (-117.9, 137.3932) centre (-119.9, 137.3932) ccw
  line L323 (-132.9, 129.3932) -> (-132.9, 118.3932)
  circle A341 centre (-115.9, 134.5432) radius 1.5
  arc A342 (-113.9, 120.6932) -> (-111.9, 118.6932) centre (-111.9, 120.6932) ccw
  arc A343 (-119.2, 116.8932) -> (-118.4, 117.6932) centre (-119.2, 117.6932) ccw construction
  line L324 (-113.4, 151.3932) -> (-113.4, 138.9932) construction
  arc A344 (-113.4, 119.9932) -> (-112.6, 119.1932) centre (-112.6, 119.9932) ccw construction
  arc A345 (-131.6, 130.8932) -> (-132.4, 130.0932) centre (-131.6, 130.0932) ccw construction
  arc A346 (-132.4, 136.6932) -> (-131.6, 135.8932) centre (-131.6, 136.6932) ccw construction
  arc A347 (-134.75, 116.2932) -> (-133.1, 114.6432) centre (-133.1, 116.2932) ccw
  arc A348 (-119.2, 135.8932) -> (-118.4, 136.6932) centre (-119.2, 136.6932) ccw construction
  arc A349 (-111.9, 133.6932) -> (-113.9, 131.6932) centre (-111.9, 131.6932) ccw
  line L325 (-134.75, 169.4932) -> (-134.75, 116.2932)
  line L326 (-113.9, 150.6932) -> (-113.9, 139.6932)
  line L327 (-134.6, 169.4932) -> (-134.6, 116.2932) construction
  line L328 (-132.4, 149.0932) -> (-132.4, 136.6932) construction
  line L329 (-117.9, 148.3932) -> (-117.9, 137.3932)
  arc A350 (-118.4, 149.0932) -> (-119.2, 149.8932) centre (-119.2, 149.0932) ccw construction
  line L330 (-118.4, 130.0932) -> (-118.4, 117.6932) construction
  arc A351 (-115.0716, 173.4432) -> (-116.5919, 172.8135) centre (-115.0716, 171.2933) ccw
  line L331 (-130.9, 116.3932) -> (-119.9, 116.3932)
  line L332 (-132.4, 130.0932) -> (-132.4, 117.6932) construction
  line L333 (-131.6, 116.8932) -> (-119.2, 116.8932) construction
  line L334 (-118.4, 149.0932) -> (-118.4, 136.6932) construction
  line L335 (-113.9, 131.6932) -> (-113.9, 120.6932)
  arc A352 (-119.0284, 170.9932) -> (-117.6142, 171.579) centre (-119.0284, 172.9932) ccw construction
  arc A353 (-119.0284, 171.1432) -> (-117.7203, 171.6851) centre (-119.0284, 172.9932) ccw
  arc A354 (-130.9, 131.3932) -> (-132.9, 129.3932) centre (-130.9, 129.3932) ccw
  arc A355 (-113.4, 138.9932) -> (-112.6, 138.1932) centre (-112.6, 138.9932) ccw construction
  arc A356 (-118.4, 168.0932) -> (-119.2, 168.8932) centre (-119.2, 168.0932) ccw construction
  arc A357 (-117.9, 148.3932) -> (-119.9, 150.3932) centre (-119.9, 148.3932) ccw
  arc A358 (-115.0716, 173.2932) -> (-116.4858, 172.7074) centre (-115.0716, 171.2933) ccw construction
  arc A359 (-119.2, 154.8932) -> (-118.4, 155.6932) centre (-119.2, 155.6932) ccw construction
  line L336 (-133.1, 170.9932) -> (-119.0284, 170.9932) construction
  arc A360 (-111.9, 152.6932) -> (-113.9, 150.6932) centre (-111.9, 150.6932) ccw
  line L337 (-130.9, 154.3932) -> (-119.9, 154.3932)
  arc A361 (-106.1426, 173.4432) -> (-104.1274, 174.2779) centre (-106.1426, 176.2932) ccw